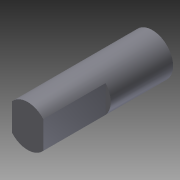
# Autodesk Inventor part: shaft
Saved by Autodesk Inventor 2012 (Build 160160000, 160)
## iProperties
Created: 2012-01-29
Part Number: shaft
Material: Steel
Document SubType Name: Modeling
Designer: Antonella Wilby
Mass: 37.8872 g
Surface Area: 17.7348 cm^2
Volume: 4.82639 cm^3
Density: 7.85 g/cm^3
Author: Antonella Wilby
Autodesk Inventor part; units mm, degrees
ref_plane "YZ Plane" through (0, 0, 0) normal (1, 0, 0) x (0, 1, 0)
ref_plane "XZ Plane" through (0, 0, 0) normal (0, 1, 0) x (-1, 0, 0)
ref_plane "XY Plane" through (0, 0, 0) normal (0, 0, 1) x (1, 0, 0)
sketch "Sketch1" plane through (0, 0, 0) normal (0, 0, 1) x (1, 0, 0)
  circle A0 centre (0, 0) radius 6.35
  dimension "d0" = 12.7
  constraints: 1 centre point, 1 coincident
  measures "d0" diameter of A0
extrude "Extrusion1" add sketch "Sketch1" along normal blind 38.1
sketch "Sketch2" plane through (0, 0, 38.1) normal (0, 0, 1) x (1, 0, 0)
  circle A0 centre (0, 0) radius 6.35 projected
  line L0 (-8.89, 0) -> (8.89, 0) projected
  line L1 (0, -8.89) -> (0, 8.89) projected
  line L2 (-4.7625, 4.2001) -> (-4.7625, -4.2001)
  line L3 (4.7625, -4.2001) -> (4.7625, 4.2001)
  arc A1 (-4.7625, -4.2001) -> (4.7625, -4.2001) centre (0, 0) ccw
  arc A2 (4.7625, 4.2001) -> (-4.7625, 4.2001) centre (0, 0) ccw
  dimension "d3" = 4.7625
  constraints: 8 point on circle, 4 end point, 3 parallel, 2 centre point, 1 coincident
  measures "d3" distance between parallel lines of L1 L3
extrude "Extrusion2" cut sketch "Sketch2" against normal blind 19.05 contours L0 L3 A0 | A0 L3 L0 | L2 L0 A0 | A0 L0 L2
body "Solid1"
